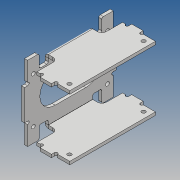
# Autodesk Inventor part: Refuerzo U
Saved by Autodesk Inventor 2017 (Build 210142000, 142)
## iProperties
Part Number: Refuerzo U
Material: Genérico
Document SubType Name: Chapa
Designer: Leo
Density: 1 g/cm^3
Appearance: Valor por defecto
Sheet Metal Rule: Por defecto
Flat Pattern Width: 19.18 cm
Flat Pattern Length: 12 cm
Flat Pattern Area: 230.16 cm^2
Sheet Metal Width: 191,800 mm
Sheet Metal Length: 120,000 mm
Sheet Metal Area: 23016,000 mm^2
Description: Aluminio compuesto routeado CNC
Author: Leo
Autodesk Inventor part; units mm, degrees
ref_plane "YZ Plane" through (0, 0, 0) normal (1, 0, 0) x (0, 1, 0)
ref_plane "XZ Plane" through (0, 0, 0) normal (0, 1, 0) x (-1, 0, 0)
ref_plane "XY Plane" through (0, 0, 0) normal (0, 0, 1) x (1, 0, 0)
sketch "Boceto1" plane through (0, 0, 0) normal (1, 0, 0) x (0, 1, 0)
  line L0 (60, 20) -> (56, 20)
  arc A0 (56, 24) -> (56, 20) centre (56, 22) ccw
  line L1 (56, 24) -> (56, 48.9)
  line L2 (-56, 48.9) -> (-56, 24)
  arc A1 (-56, 20) -> (-56, 24) centre (-56, 22) ccw
  line L3 (-56, 20) -> (-60, 20)
  line L4 (-60, 20) -> (-60, -20)
  line L5 (-60, -20) -> (-56, -20)
  arc A2 (-56, -24) -> (-56, -20) centre (-56, -22) ccw
  line L6 (-56, -24) -> (-56, -48.9)
  line L7 (56, -48.9) -> (56, -24)
  arc A3 (56, -20) -> (56, -24) centre (56, -22) ccw
  line L8 (56, -20) -> (60, -20)
  line L9 (60, -20) -> (60, 20)
  line L10 (56, 48.9) -> (43, 48.9)
  line L11 (60, 0) -> (-60, 0) construction
  line L12 (41, 46.9) -> (41, 33.9)
  line L13 (56, 52.9) -> (56, 56.9)
  arc A4 (56, 60.9) -> (56, 56.9) centre (56, 58.9) ccw
  line L14 (56, 60.9) -> (60, 60.9)
  line L15 (60, 60.9) -> (60, 75.9)
  line L16 (60, 75.9) -> (56, 75.9)
  arc A5 (56, 79.9) -> (56, 75.9) centre (56, 77.9) ccw
  line L17 (56, 79.9) -> (56, 95.9)
  line L18 (56, 95.9) -> (-56, 95.9)
  line L19 (-56, 95.9) -> (-56, 79.9)
  arc A6 (43, 48.9) -> (41, 46.9) centre (43, 46.9) ccw
  line L20 (56, 52.9) -> (35, 52.9)
  arc A7 (35, 52.9) -> (29, 46.9) centre (35, 46.9) ccw
  line L21 (29, 46.9) -> (29, 33.9)
  arc A8 (-56, 75.9) -> (-56, 79.9) centre (-56, 77.9) ccw
  line L22 (-56, 75.9) -> (-60, 75.9)
  line L23 (-60, 75.9) -> (-60, 60.9)
  line L24 (-60, 60.9) -> (-56, 60.9)
  arc A9 (-56, 56.9) -> (-56, 60.9) centre (-56, 58.9) ccw
  line L25 (-56, 56.9) -> (-56, 52.9)
  line L26 (-56, 52.9) -> (-35, 52.9)
  arc A10 (-29, 46.9) -> (-35, 52.9) centre (-35, 46.9) ccw
  line L27 (-29, 46.9) -> (-29, 33.9)
  line L28 (-41, 33.9) -> (-41, 46.9)
  arc A11 (-41, 46.9) -> (-43, 48.9) centre (-43, 46.9) ccw
  line L29 (-43, 48.9) -> (-56, 48.9)
  line L30 (0, 46.6797) -> (0, -46.6797) construction
  line L31 (56, -48.9) -> (43, -48.9)
  line L32 (41, -46.9) -> (41, -33.9)
  line L33 (56, -52.9) -> (56, -56.9)
  arc A12 (56, -56.9) -> (56, -60.9) centre (56, -58.9) ccw
  line L34 (56, -60.9) -> (60, -60.9)
  line L35 (60, -60.9) -> (60, -75.9)
  line L36 (60, -75.9) -> (56, -75.9)
  arc A13 (56, -75.9) -> (56, -79.9) centre (56, -77.9) ccw
  line L37 (56, -79.9) -> (56, -95.9)
  line L38 (56, -95.9) -> (-56, -95.9)
  line L39 (-56, -95.9) -> (-56, -79.9)
  arc A14 (41, -46.9) -> (43, -48.9) centre (43, -46.9) ccw
  line L40 (56, -52.9) -> (35, -52.9)
  arc A15 (29, -46.9) -> (35, -52.9) centre (35, -46.9) ccw
  line L41 (29, -46.9) -> (29, -33.9)
  arc A16 (-56, -79.9) -> (-56, -75.9) centre (-56, -77.9) ccw
  line L42 (-56, -75.9) -> (-60, -75.9)
  line L43 (-60, -75.9) -> (-60, -60.9)
  line L44 (-60, -60.9) -> (-56, -60.9)
  arc A17 (-56, -60.9) -> (-56, -56.9) centre (-56, -58.9) ccw
  line L45 (-56, -56.9) -> (-56, -52.9)
  line L46 (-56, -52.9) -> (-35, -52.9)
  arc A18 (-35, -52.9) -> (-29, -46.9) centre (-35, -46.9) ccw
  line L47 (-29, -46.9) -> (-29, -33.9)
  line L48 (-41, -33.9) -> (-41, -46.9)
  arc A19 (-43, -48.9) -> (-41, -46.9) centre (-43, -46.9) ccw
  line L49 (-43, -48.9) -> (-56, -48.9)
  line L50 (-29, 37.9) -> (29, 37.9) construction
  line L51 (-29, -37.9) -> (29, -37.9) construction
  circle A20 centre (48.5, 87.9) radius 2.5
  circle A21 centre (-48.5, 87.9) radius 2.5
  circle A22 centre (48.5, 30) radius 2.5
  circle A23 centre (-48.5, 30) radius 2.5
  line L52 (20, 20) -> (-20, 20)
  arc A24 (-20, 20) -> (-20, -20) centre (-20, 0) ccw
  line L53 (-20, -20) -> (20, -20)
  arc A25 (20, -20) -> (20, 20) centre (20, 0) ccw
  circle A26 centre (48.5, -87.9) radius 2.5
  circle A27 centre (-48.5, -87.9) radius 2.5
  circle A28 centre (48.5, -30) radius 2.5
  circle A29 centre (-48.5, -30) radius 2.5
  arc A30 (39, 31.9) -> (41, 33.9) centre (39, 33.9) ccw
  line L54 (39, 31.9) -> (31, 31.9)
  arc A31 (29, 33.9) -> (31, 31.9) centre (31, 33.9) ccw
  arc A32 (-41, 33.9) -> (-39, 31.9) centre (-39, 33.9) ccw
  line L55 (-39, 31.9) -> (-31, 31.9)
  arc A33 (-31, 31.9) -> (-29, 33.9) centre (-31, 33.9) ccw
  arc A34 (41, -33.9) -> (39, -31.9) centre (39, -33.9) ccw
  line L56 (39, -31.9) -> (31, -31.9)
  arc A35 (31, -31.9) -> (29, -33.9) centre (31, -33.9) ccw
  arc A36 (-39, -31.9) -> (-41, -33.9) centre (-39, -33.9) ccw
  line L57 (-39, -31.9) -> (-31, -31.9)
  arc A37 (-29, -33.9) -> (-31, -31.9) centre (-31, -33.9) ccw
  point P0 (0, 0)
  point P1 (0, 0)
  point P2 (0, 20)
  dimension "d0" = 4
  dimension "d1" = 40
  dimension "d2" = 2
  dimension "d5" = 2
  dimension "d9" = 15
  dimension "d10" = 20
  dimension "d11" = 75.8
  dimension "d13" = 120
  dimension "d14" = 58
  dimension "d15" = 23
  dimension "d16" = 4
  dimension "d31" = 8
  dimension "d32" = 7.5
  dimension "d33" = 15
  dimension "d34" = 5
  dimension "d35" = 10
  dimension "d36" = 7.5
  dimension "d37" = 40
  dimension "d38" = 20
  dimension "d39" = 12
  dimension "d40" = 4
  dimension "d41" = 6
  dimension "d42" = 2
  dimension "d43" = 6
  constraints: 116 end point, 60 point on circle, 44 symmetric about line, 38 centre point, 33 tangent, 24 point on line, 16 perpendicular, 10 horizontal, 9 equal radius, 8 vertical, 5 midpoint, 4 equal length, 2 collinear, 2 horizontal alignment, 2 vertical alignment, 1 coincident, 31 other
  measures "d0" distance between parallel lines of L1 L9
  measures "d1" distance of L8.end L0.start
  measures "d2" radius of A3
  measures "d5" radius of A6
  measures "d9" distance of L14.end L15.end
  measures "d10" distance between parallel lines of L16 L18
  measures "d11" diameter of L50 L11
  measures "d13" distance between parallel lines of L4 L9
  measures "d14" distance between parallel lines of L27 L21
  measures "d15" distance between parallel lines of L14 L50
  measures "d16" distance of L13.start L13.end
  measures "d31" distance from line of L18 A20.centre
  measures "d32" distance from line of L17 A20.centre
  measures "d33" distance between parallel lines of L12 L1
  measures "d34" diameter of A20
  measures "d35" distance from line of A22.centre L0
  measures "d36" distance from line of L19 A21.centre
  measures "d37" distance between parallel lines of L53 L52
  measures "d38" distance edge to line of A25 L9
  measures "d39" distance between parallel lines of L21 L12
  measures "d40" distance between parallel lines of L20 L10
  measures "d41" distance between parallel lines of L50 L54
  measures "d42" radius of A30
  measures "d43" radius of A7
extrude "Extrusión1" add sketch "Boceto1" against normal blind 4
fold "Pliegue1" angle 90 bend radius 0.1 thickness 4 k factor 0.44 line from (0, -29, 37.9) to (0, 29, 37.9) line at bend start moving side (0, 0, 1) folds toward (1, 0, 0)
fold "Pliegue2" angle 90 bend radius 0.1 thickness 4 k factor 0.44 line from (0, -29, -37.9) to (0, 29, -37.9) line at bend start moving side (0, 0, -1) folds toward (1, 0, 0)
equation "\"d32\" = 0.5 * d33"
equation "\"d36\" = d32"
equation "\"d40\" = d16"
equation "\"d19\" = Anchura_desahogo_plegado"
equation "\"d20\" = Profundidad_desahogo_plegado"
equation "\"d21\" = Remanente_mínimo"
equation "\"d22\" = Radio_pliegue"
equation "\"d25\" = Anchura_desahogo_plegado"
equation "\"d26\" = Profundidad_desahogo_plegado"
equation "\"d27\" = Remanente_mínimo"
equation "\"d28\" = Radio_pliegue"
equation "\"Radio_pliegue\" = Grosor"
equation "\"Anchura_desahogo_plegado\" = Grosor"
equation "\"Profundidad_desahogo_plegado\" = 0.5 * Grosor"
equation "\"Tamaño_destalonado\" = 4 * Grosor"
equation "\"Remanente_mínimo\" = 2 * Grosor"
equation "\"Radiodetransición\" = Radio_pliegue"
equation "\"Tamaño_de_radio_de_Jacobi\" = Grosor"
equation "\"TamañoSeparación\" = Grosor"
equation "\"Grosor\" = 4"
